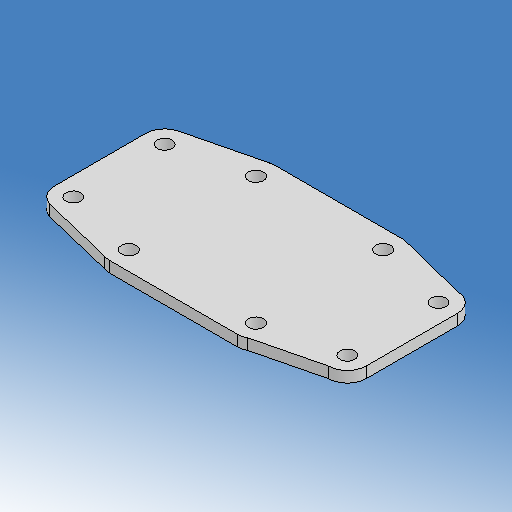
# Autodesk Inventor part: LidarMountAdapter
Saved by Autodesk Inventor 2025 (Build 290162000, 162)
## iProperties
Created: 2024-06-15
Part Number: LidarMountAdapter
Material: Generic
Document SubType Name: Sheet Metal
Designer: seene
Density: 1 g/cm^3
Sheet Metal Rule: Default
Appearance: Default
Author: seene
Autodesk Inventor part; units mm, degrees
ref_plane "YZ Plane" through (0, 0, 0) normal (1, 0, 0) x (0, 1, 0)
ref_plane "XZ Plane" through (0, 0, 0) normal (0, 1, 0) x (-1, 0, 0)
ref_plane "XY Plane" through (0, 0, 0) normal (0, 0, 1) x (1, 0, 0)
sketch "Sketch1" plane through (0, 0, 0) normal (0, 1, 0) x (-1, 0, 0)
  line L0 (-43.3451, -30.2749) -> (43.3451, -30.2749)
  line L1 (43.3451, -30.2749) -> (43.3451, 30.2749)
  line L2 (43.3451, 30.2749) -> (-43.3451, 30.2749)
  line L3 (-43.3451, 30.2749) -> (-43.3451, -30.2749)
  line L4 (-43.3451, -30.2749) -> (43.3451, 30.2749) construction
  line L5 (43.3451, -30.2749) -> (-43.3451, 30.2749) construction
  circle A0 centre (0, 0) radius 25 construction
  circle A1 centre (17.6777, -17.6777) radius 2.1
  circle A2 centre (17.6777, 17.6777) radius 2.1
  circle A3 centre (-17.6777, 17.6777) radius 2.1
  circle A4 centre (-17.6777, -17.6777) radius 2.1
  line L6 (25.4, -25.4) -> (-25.4, -25.4) construction
  line L7 (-25.4, -25.4) -> (-25.4, 25.4) construction
  line L8 (-25.4, 25.4) -> (25.4, 25.4) construction
  line L9 (25.4, 25.4) -> (25.4, -25.4) construction
  line L10 (25.4, -25.4) -> (-25.4, 25.4) construction
  line L11 (25.4, 25.4) -> (-25.4, -25.4) construction
  circle A5 centre (38.1, -12.7) radius 2.0701
  circle A6 centre (38.1, 12.7) radius 2.0701
  circle A7 centre (-38.1, 12.7) radius 2.0701
  circle A8 centre (-38.1, -12.7) radius 2.0701
  circle A9 centre (38.1, -12.7) radius 5.2451
  circle A10 centre (-38.1, -12.7) radius 5.2451
  circle A11 centre (38.1, 12.7) radius 5.2451
  circle A12 centre (-38.1, 12.7) radius 5.2451
  circle A13 centre (17.6777, -17.6777) radius 5.275
  circle A14 centre (-17.6777, -17.6777) radius 5.275
  circle A15 centre (17.6777, 17.6777) radius 5.275
  circle A16 centre (-17.6777, 17.6777) radius 5.275
  line L12 (39.7534, 17.6777) -> (19.6427, 22.573)
  line L13 (-20.1088, 22.3591) -> (-38.1, 17.9451)
  line L14 (39.2127, -17.8257) -> (18.9346, -22.8007)
  line L15 (-18.9732, -22.7911) -> (-38.1, -17.9451)
  line L16 (17.6777, 22.9527) -> (-17.6777, 22.9527)
  line L17 (17.6777, -22.9527) -> (-17.6777, -22.9527)
  point P0 (0, 0)
  point P1 (39.7131, 17.6909)
  point P2 (-39.7172, 17.6896)
  point P3 (-39.7131, -17.6909)
  point P4 (39.7172, -17.6896)
  point P5 (-43.3451, -12.7)
  point P6 (43.3451, -12.7)
  point P7 (43.3451, 12.7)
  point P8 (-43.3451, 12.7)
  dimension "d7" = 50
  dimension "d2" = 360
  dimension "d4" = 4.2
  dimension "d29" = 50.8
  dimension "d30" = 50.8
  dimension "d31" = 4.1402
  dimension "d32" = 4.1402
  dimension "d33" = 12.7
  dimension "d36" = 360
  dimension "d39" = 25.4
  dimension "d40" = 12.7
  dimension "d41" = 3.175
  dimension "d43" = 3.175
  dimension "d45" = 3.175
  dimension "d46" = 3.175
  dimension "d47" = 3.175
  dimension "d48" = 3.175
  dimension "d49" = 3.175
  dimension "d50" = 3.175
  measures "d4" diameter of A1
  measures "d29" distance of L7.end L8.end
  measures "d30" distance of L6.end L7.end
  measures "d31" diameter of A5
  measures "d32" diameter of A6
  measures "d33" distance from line of L9 A5.centre
  measures "d39" distance of A6.centre A5.centre
  measures "d40" vertical distance of point (0, 0) A5.centre
  measures "d41" radial gap between concentric circles of A5 A9
  measures "d43" radial gap between concentric circles of A8 A10
  measures "d45" radial gap between concentric circles of A6 A11
  measures "d46" radial gap between concentric circles of A7 A12
  measures "d47" radial gap between concentric circles of A1 A13
  measures "d49" radial gap between concentric circles of A2 A15
  measures "d50" radial gap between concentric circles of A3 A16
extrude "Plate1" add sketch "Sketch1" along normal blind 3.048 contours L3 A12 L13 A16 L16 A15 L12 A11 L1 A9 L14 A13 L17 A14 L15 A10 | A10 | A9 | A12 | A11 L12 | A14 | A13 | A16 | A15 picked at (42.2152, 12.1134)
equation "\"d8\" = Thickness"
equation "\"d40\" = 0.5 * d39"
equation "\"BendRadius\" = Thickness"
equation "\"BendReliefWidth\" = Thickness"
equation "\"BendReliefDepth\" = 0.5 * Thickness"
equation "\"CornerReliefSize\" = 4 * Thickness"
equation "\"MinimumRemnant\" = 2 * Thickness"
equation "\"TransitionRadius\" = BendRadius"
equation "\"JacobiRadiusSize\" = BendRadius"
equation "\"GapSize\" = Thickness"
equation "\"Thickness\" = 3.048"
body "Solid1"
